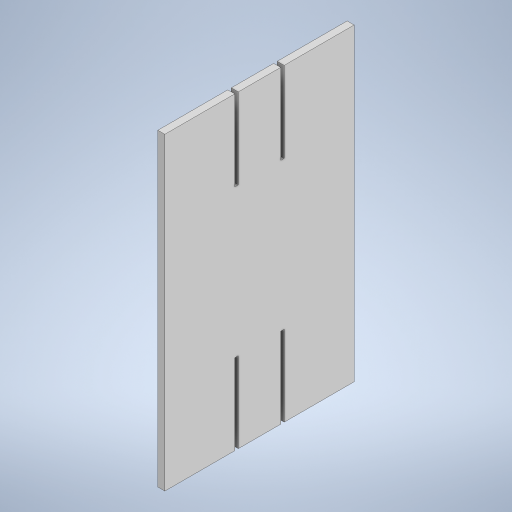
# Autodesk Inventor part: 4x2020_raw
Saved by Autodesk Inventor 2024 (Build 280153000, 153)
## iProperties
Created: 2025-12-30
Part Number: 4x2020_raw
Material: Generic
Document SubType Name: Modeling
Designer: schar
Density: 1 g/cm^3
Appearance: Default
Author: schar
d0: 88,300 mm
d1: 54,112 mm
d2: 20,000 mm
d3: 20,000 mm
d4: 1,000 mm
d5: 20,000 mm
d6: 20,000 mm
d7: 1,000 mm
d8: 20,000 mm
d9: 20,000 mm
d10: 20,000 mm
d11: 20,000 mm
d12: 1,000 mm
d13: 1,000 mm
d14: 3,000 mm
d15: 3,000 mm
d16: 3,000 mm
d17: 3,000 mm
Autodesk Inventor part; units mm, degrees
ref_plane "YZ Plane" through (0, 0, 0) normal (1, 0, 0) x (0, 1, 0)
ref_plane "XZ Plane" through (0, 0, 0) normal (0, 1, 0) x (-1, 0, 0)
ref_plane "XY Plane" through (0, 0, 0) normal (0, 0, 1) x (1, 0, 0)
sketch "Sketch1" plane through (0, 0, 0) normal (1, 0, 0) x (0, 1, 0)
  line L0 (44.15, 27.056) -> (-44.15, 27.056)
  line L1 (-44.15, 27.056) -> (-44.15, -27.056)
  line L2 (-44.15, -27.056) -> (44.15, -27.056)
  line L3 (44.15, -27.056) -> (44.15, 27.056)
  line L4 (44.15, 27.056) -> (-44.15, -27.056) construction
  line L5 (-44.15, 27.056) -> (44.15, -27.056) construction
  line L6 (44.15, 27.056) -> (24.15, 27.056)
  line L7 (24.15, 27.056) -> (24.15, 7.056)
  line L8 (24.15, 7.056) -> (44.15, 7.056)
  line L9 (44.15, 7.056) -> (44.15, 27.056)
  line L10 (24.15, 7.056) -> (24.15, 6.056)
  line L11 (24.15, 6.056) -> (44.15, 6.056)
  line L12 (44.15, -27.056) -> (24.15, -27.056)
  line L13 (24.15, -27.056) -> (24.15, -7.056)
  line L14 (24.15, -7.056) -> (44.15, -7.056)
  line L15 (44.15, -7.056) -> (44.15, -27.056)
  line L16 (24.15, -7.056) -> (24.15, -6.056)
  line L17 (24.15, -6.056) -> (44.15, -6.056)
  line L18 (-44.15, 27.056) -> (-24.15, 27.056)
  line L19 (-24.15, 27.056) -> (-24.15, 7.056)
  line L20 (-24.15, 7.056) -> (-44.15, 7.056)
  line L21 (-44.15, 7.056) -> (-44.15, 27.056)
  line L22 (-44.15, -27.056) -> (-24.15, -27.056)
  line L23 (-24.15, -27.056) -> (-24.15, -7.056)
  line L24 (-24.15, -7.056) -> (-44.15, -7.056)
  line L25 (-44.15, -7.056) -> (-44.15, -27.056)
  line L26 (-24.15, 7.056) -> (-24.15, 6.056)
  line L27 (-24.15, 6.056) -> (-44.15, 6.056)
  line L28 (-24.15, -7.056) -> (-24.15, -6.056)
  line L29 (-24.15, -6.056) -> (-44.15, -6.056)
  line L30 (24.15, 7.056) -> (21.15, 7.056)
  line L31 (21.15, 7.056) -> (21.15, 6.056)
  line L32 (21.15, 6.056) -> (24.15, 6.056)
  line L33 (24.15, 6.056) -> (24.15, 7.056)
  line L34 (24.15, -6.056) -> (21.15, -6.056)
  line L35 (21.15, -6.056) -> (21.15, -7.056)
  line L36 (21.15, -7.056) -> (24.15, -7.056)
  line L37 (24.15, -7.056) -> (24.15, -6.056)
  line L38 (-24.15, -6.056) -> (-21.15, -6.056)
  line L39 (-21.15, -6.056) -> (-21.15, -7.056)
  line L40 (-21.15, -7.056) -> (-24.15, -7.056)
  line L41 (-24.15, -7.056) -> (-24.15, -6.056)
  line L42 (-24.15, 7.056) -> (-21.15, 7.056)
  line L43 (-21.15, 7.056) -> (-21.15, 6.056)
  line L44 (-21.15, 6.056) -> (-24.15, 6.056)
  line L45 (-24.15, 6.056) -> (-24.15, 7.056)
  point P0 (0, 0)
  point P1 (0, 0)
  dimension "d0" = 88.3
  dimension "d1" = 54.112
  dimension "d2" = 20
  dimension "d3" = 20
  dimension "d4" = 1
  dimension "d5" = 20
  dimension "d6" = 20
  dimension "d7" = 1
  dimension "d8" = 20
  dimension "d9" = 20
  dimension "d10" = 20
  dimension "d11" = 20
  dimension "d12" = 1
  dimension "d13" = 1
  dimension "d14" = 3
  dimension "d15" = 3
  dimension "d16" = 3
  dimension "d17" = 3
  constraints: 92 end point, 19 parallel, 13 perpendicular, 9 horizontal, 4 point on line, 3 vertical, 2 midpoint
  measures "d0" distance of L2.end L2.start
  measures "d1" distance of L2.start L5.start
  measures "d2" distance of L8.end L30.start
  measures "d3" distance of L30.start L6.end
  measures "d4" distance of L30.start L11.start
  measures "d5" distance of L16.start L14.end
  measures "d6" distance of L13.start L16.start
  measures "d7" distance of L16.start L34.start
  measures "d8" distance of L42.start L20.end
  measures "d9" distance of L19.start L42.start
  measures "d10" distance of L24.end L24.start
  measures "d11" distance of L24.start L22.end
  measures "d12" distance of L42.start L27.start
  measures "d13" distance of L24.start L29.start
  measures "d14" distance of L32.end L32.start
  measures "d15" distance of L36.end L35.end
  measures "d16" distance of L40.start L41.start
  measures "d17" distance of L44.start L44.end
extrude "Extrusion1" add sketch "Sketch1" along normal blind 2 contours L3 L8 L7 L0 | L7 L30 L31 L32 L11 L3 L17 L34 L35 L36 L13 L2 L23 L40 L39 L38 L29 L1 L27 L44 L43 L42 L19 L0 | L19 L20 L1 L0 | L3 L2 L13 L14 | L24 L23 L2 L1
body "Solid1"
